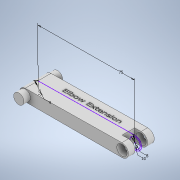
# Autodesk Inventor part: Elbow extension
Saved by Autodesk Inventor 2020 (Build 240168000, 168)
## iProperties
Created: 2020-12-23
Part Number: Elbow extension
Material: Generic
Document SubType Name: Modeling
Designer: frost
Density: 1 g/cm^3
Appearance: Default
Author: frost
Autodesk Inventor part; units mm, degrees
ref_plane "YZ Plane" through (0, 0, 0) normal (1, 0, 0) x (0, 1, 0)
ref_plane "XZ Plane" through (0, 0, 0) normal (0, 1, 0) x (-1, 0, 0)
ref_plane "XY Plane" through (0, 0, 0) normal (0, 0, 1) x (1, 0, 0)
sketch "Sketch1" plane through (0, 0, 0) normal (0, 0, 1) x (1, 0, 0)
  circle A0 centre (0, 0) radius 4
  circle A1 centre (74.9981, 0.5286) radius 4
  arc A2 (-0.0617, 4.4996) -> (0.0017, -4.5) centre (0, 0) ccw
  arc A3 (75, -4.4714) -> (74.9296, 5.5281) centre (74.9981, 0.5286) ccw
  line L0 (-0.0617, 4.4996) -> (74.9296, 5.5281)
  line L1 (0.0017, -4.5) -> (75, -4.4714)
  dimension "d0" = 8
  dimension "d1" = 8
  dimension "d2" = 75
  dimension "d3" = 9
  dimension "d4" = 10
  constraints: 4 centre point, 4 end point, 4 point on circle, 4 tangent, 3 coincident
  measures "d0" diameter of A0
  measures "d1" diameter of A1
  measures "d2" distance of A1.centre A0.centre
  measures "d3" diameter of A2
  measures "d4" diameter of A3
extrude "Extrusion1" add sketch "Sketch1" along normal mid plane 20 contours A0 | A1 | L0 A3 L1 A2
extrude "Extrusion2" add sketch "Sketch1" along normal mid plane 30 contours A0
extrude "Extrusion3" cut sketch "Sketch1" along normal mid plane 30 contours A1
sketch "Sketch2" plane through (-0.0617, 4.4996, 10) normal (-0.0137142, 0.999906, 0) x (0.999906, 0.0137142, 0)
  line L0 (15.9596, 15.3498) -> (61.2005, 15.3498) construction
  line L1 (61.2005, 15.3498) -> (61.2005, 12.0996) construction
  line L2 (61.2005, 12.0996) -> (15.9596, 12.0996) construction
  line L3 (15.9596, 12.0996) -> (15.9596, 15.3498) construction
  line L4 (16.4243, 12.1638) -> (16.4243, 15.2138)
  line L5 (16.4243, 15.2138) -> (19.2865, 15.2138)
  line L6 (19.2865, 15.2138) -> (19.2865, 14.853)
  line L7 (19.2865, 14.853) -> (17.0323, 14.853)
  line L8 (17.0323, 14.853) -> (17.0323, 14.0176)
  line L9 (17.0323, 14.0176) -> (19.1332, 14.0176)
  line L10 (19.1332, 14.0176) -> (19.1332, 13.6567)
  line L11 (19.1332, 13.6567) -> (17.0323, 13.6567)
  line L12 (17.0323, 13.6567) -> (17.0323, 12.5247)
  line L13 (17.0323, 12.5247) -> (19.2865, 12.5247)
  line L14 (19.2865, 12.5247) -> (19.2865, 12.1638)
  line L15 (19.2865, 12.1638) -> (16.4243, 12.1638)
  line L16 (20.4976, 12.1638) -> (19.9192, 12.1638)
  line L17 (19.9192, 12.1638) -> (19.9192, 15.3498)
  line L18 (19.9192, 15.3498) -> (20.4976, 15.3498)
  line L19 (20.4976, 15.3498) -> (20.4976, 12.1638)
  spline S0 degree 2 poles (24.2248, 13.3453) (24.2248, 12.7842) (23.4067, 12.0996) (22.7937, 12.0996) knots 0 0 0 1 2 2 2
  spline S1 degree 2 poles (22.7937, 12.0996) (22.5144, 12.0996) (22.1165, 12.191) (21.9237, 12.2701) knots 0 0 0 1 2 2 2
  line L20 (21.9237, 12.2701) -> (21.8866, 12.1638)
  line L21 (21.8866, 12.1638) -> (21.3453, 12.1638)
  line L22 (21.3453, 12.1638) -> (21.3453, 15.3498)
  line L23 (21.3453, 15.3498) -> (21.9237, 15.3498)
  line L24 (21.9237, 15.3498) -> (21.9237, 14.2128)
  spline S2 degree 2 poles (21.9237, 14.2128) (22.1412, 14.3438) (22.6528, 14.5168) (22.9741, 14.5168) knots 0 0 0 1 2 2 2
  spline S3 degree 2 poles (22.9741, 14.5168) (23.555, 14.5168) (24.2248, 13.8965) (24.2248, 13.3453) knots 0 0 0 1 2 2 2
  spline S4 degree 2 poles (23.6291, 13.3156) (23.6291, 13.7259) (23.2534, 14.151) (22.8382, 14.151) knots 0 0 0 1 2 2 2
  spline S5 degree 2 poles (22.8382, 14.151) (22.6034, 14.151) (22.1214, 14.0027) (21.9237, 13.889) knots 0 0 0 1 2 2 2
  line L25 (21.9237, 13.889) -> (21.9237, 12.5766)
  spline S6 degree 2 poles (21.9237, 12.5766) (22.1412, 12.5049) (22.4798, 12.4456) (22.6825, 12.4456) knots 0 0 0 1 2 2 2
  spline S7 degree 2 poles (22.6825, 12.4456) (23.1249, 12.4456) (23.6291, 12.8633) (23.6291, 13.3156) knots 0 0 0 1 2 2 2
  spline S8 degree 2 poles (27.6455, 13.3082) (27.6455, 12.7298) (26.8101, 12.0996) (26.1156, 12.0996) knots 0 0 0 1 2 2 2
  spline S9 degree 2 poles (26.1156, 12.0996) (25.4013, 12.0996) (24.5807, 12.7496) (24.5807, 13.3082) knots 0 0 0 1 2 2 2
  spline S10 degree 2 poles (24.5807, 13.3082) (24.5807, 13.8816) (25.426, 14.5168) (26.1156, 14.5168) knots 0 0 0 1 2 2 2
  spline S11 degree 2 poles (26.1156, 14.5168) (26.8101, 14.5168) (27.6455, 13.8841) (27.6455, 13.3082) knots 0 0 0 1 2 2 2
  spline S12 degree 2 poles (27.0499, 13.3082) (27.0499, 13.7531) (26.5654, 14.1856) (26.1156, 14.1856) knots 0 0 0 1 2 2 2
  spline S13 degree 2 poles (26.1156, 14.1856) (25.6658, 14.1856) (25.1764, 13.7531) (25.1764, 13.3082) knots 0 0 0 1 2 2 2
  spline S14 degree 2 poles (25.1764, 13.3082) (25.1764, 12.8757) (25.6658, 12.4308) (26.1156, 12.4308) knots 0 0 0 1 2 2 2
  spline S15 degree 2 poles (26.1156, 12.4308) (26.5605, 12.4308) (27.0499, 12.8683) (27.0499, 13.3082) knots 0 0 0 1 2 2 2
  line L26 (32.401, 14.4526) -> (31.531, 12.1638)
  line L27 (31.531, 12.1638) -> (30.9971, 12.1638)
  line L28 (30.9971, 12.1638) -> (30.1567, 13.9286)
  line L29 (30.1567, 13.9286) -> (29.3238, 12.1638)
  line L30 (29.3238, 12.1638) -> (28.7924, 12.1638)
  line L31 (28.7924, 12.1638) -> (27.9125, 14.4526)
  line L32 (27.9125, 14.4526) -> (28.5131, 14.4526)
  line L33 (28.5131, 14.4526) -> (29.1211, 12.6804)
  line L34 (29.1211, 12.6804) -> (29.9343, 14.4526)
  line L35 (29.9343, 14.4526) -> (30.4113, 14.4526)
  line L36 (30.4113, 14.4526) -> (31.2492, 12.6804)
  line L37 (31.2492, 12.6804) -> (31.8201, 14.4526)
  line L38 (31.8201, 14.4526) -> (32.401, 14.4526)
  line L39 (34.922, 12.1638) -> (34.922, 15.2138)
  line L40 (34.922, 15.2138) -> (37.7842, 15.2138)
  line L41 (37.7842, 15.2138) -> (37.7842, 14.853)
  line L42 (37.7842, 14.853) -> (35.5301, 14.853)
  line L43 (35.5301, 14.853) -> (35.5301, 14.0176)
  line L44 (35.5301, 14.0176) -> (37.631, 14.0176)
  line L45 (37.631, 14.0176) -> (37.631, 13.6567)
  line L46 (37.631, 13.6567) -> (35.5301, 13.6567)
  line L47 (35.5301, 13.6567) -> (35.5301, 12.5247)
  line L48 (35.5301, 12.5247) -> (37.7842, 12.5247)
  line L49 (37.7842, 12.5247) -> (37.7842, 12.1638)
  line L50 (37.7842, 12.1638) -> (34.922, 12.1638)
  line L51 (41.0739, 12.1638) -> (40.3646, 12.1638)
  line L52 (40.3646, 12.1638) -> (39.5292, 13.0264)
  line L53 (39.5292, 13.0264) -> (38.6715, 12.1638)
  line L54 (38.6715, 12.1638) -> (38.0165, 12.1638)
  line L55 (38.0165, 12.1638) -> (39.2079, 13.2983)
  line L56 (39.2079, 13.2983) -> (38.0289, 14.4526)
  line L57 (38.0289, 14.4526) -> (38.7383, 14.4526)
  line L58 (38.7383, 14.4526) -> (39.5662, 13.5949)
  line L59 (39.5662, 13.5949) -> (40.419, 14.4526)
  line L60 (40.419, 14.4526) -> (41.0739, 14.4526)
  line L61 (41.0739, 14.4526) -> (39.89, 13.3255)
  line L62 (39.89, 13.3255) -> (41.0739, 12.1638)
  spline S16 degree 2 poles (42.5569, 12.1194) (42.0848, 12.1194) (41.5559, 12.4777) (41.5559, 12.8658) knots 0 0 0 1 2 2 2
  line L63 (41.5559, 12.8658) -> (41.5559, 14.1337)
  line L64 (41.5559, 14.1337) -> (41.1654, 14.1337)
  line L65 (41.1654, 14.1337) -> (41.1654, 14.4526)
  line L66 (41.1654, 14.4526) -> (41.5559, 14.4526)
  line L67 (41.5559, 14.4526) -> (41.5559, 15.11)
  line L68 (41.5559, 15.11) -> (42.1343, 15.11)
  line L69 (42.1343, 15.11) -> (42.1343, 14.4526)
  line L70 (42.1343, 14.4526) -> (43.1971, 14.4526)
  line L71 (43.1971, 14.4526) -> (43.1971, 14.1337)
  line L72 (43.1971, 14.1337) -> (42.1343, 14.1337)
  line L73 (42.1343, 14.1337) -> (42.1343, 13.0437)
  spline S17 degree 2 poles (42.1343, 13.0437) (42.1343, 12.8707) (42.1516, 12.6804) (42.2134, 12.5988) knots 0 0 0 1 2 2 2
  spline S18 degree 2 poles (42.2134, 12.5988) (42.2653, 12.5272) (42.5001, 12.4555) (42.7003, 12.4555) knots 0 0 0 1 2 2 2
  spline S19 degree 2 poles (42.7003, 12.4555) (42.8412, 12.4555) (43.1056, 12.5123) (43.1625, 12.5296) knots 0 0 0 1 2 2 2
  line L74 (43.1625, 12.5296) -> (43.1971, 12.5296)
  line L75 (43.1971, 12.5296) -> (43.1971, 12.1836)
  spline S20 degree 2 poles (43.1971, 12.1836) (43.034, 12.154) (42.7003, 12.1194) (42.5569, 12.1194) knots 0 0 0 1 2 2 2
  spline S21 degree 2 poles (45.1151, 12.1119) (44.2945, 12.1119) (43.3874, 12.7274) (43.3874, 13.2958) knots 0 0 0 1 2 2 2
  spline S22 degree 2 poles (43.3874, 13.2958) (43.3874, 13.8544) (44.2673, 14.5168) (44.9767, 14.5168) knots 0 0 0 1 2 2 2
  spline S23 degree 2 poles (44.9767, 14.5168) (45.2955, 14.5168) (45.7874, 14.3933) (45.9727, 14.2623) knots 0 0 0 1 2 2 2
  spline S24 degree 2 poles (45.9727, 14.2623) (46.1556, 14.1313) (46.3534, 13.7531) (46.3534, 13.4788) knots 0 0 0 1 2 2 2
  line L76 (46.3534, 13.4788) -> (46.3534, 13.2687)
  line L77 (46.3534, 13.2687) -> (43.9732, 13.2687)
  spline S25 degree 2 poles (43.9732, 13.2687) (43.9732, 12.8707) (44.5763, 12.4481) (45.1077, 12.4481) knots 0 0 0 1 2 2 2
  spline S26 degree 2 poles (45.1077, 12.4481) (45.298, 12.4481) (45.6638, 12.5049) (45.8121, 12.5494) knots 0 0 0 1 2 2 2
  spline S27 degree 2 poles (45.8121, 12.5494) (45.9703, 12.5988) (46.1853, 12.6854) (46.2545, 12.7249) knots 0 0 0 1 2 2 2
  line L78 (46.2545, 12.7249) -> (46.2891, 12.7249)
  line L79 (46.2891, 12.7249) -> (46.2891, 12.3047)
  spline S28 degree 2 poles (46.2891, 12.3047) (46.1878, 12.2775) (45.8862, 12.1984) (45.7676, 12.1762) knots 0 0 0 1 2 2 2
  spline S29 degree 2 poles (45.7676, 12.1762) (45.597, 12.1441) (45.3252, 12.1119) (45.1151, 12.1119) knots 0 0 0 1 2 2 2
  spline S30 degree 2 poles (45.7898, 13.5628) (45.7849, 13.7185) (45.686, 13.9459) (45.5921, 14.0225) knots 0 0 0 1 2 2 2
  spline S31 degree 2 poles (45.5921, 14.0225) (45.4908, 14.109) (45.1744, 14.2005) (44.9421, 14.2005) knots 0 0 0 1 2 2 2
  spline S32 degree 2 poles (44.9421, 14.2005) (44.7097, 14.2005) (44.3884, 14.109) (44.2549, 14.02) knots 0 0 0 1 2 2 2
  spline S33 degree 2 poles (44.2549, 14.02) (44.1264, 13.9286) (43.9905, 13.7086) (43.9732, 13.5628) knots 0 0 0 1 2 2 2
  line L80 (43.9732, 13.5628) -> (45.7898, 13.5628)
  line L81 (49.6357, 12.1638) -> (49.0573, 12.1638)
  line L82 (49.0573, 12.1638) -> (49.0573, 13.4689)
  spline S34 degree 2 poles (49.0573, 13.4689) (49.0573, 13.627) (49.0104, 13.8989) (48.9461, 13.9805) knots 0 0 0 1 2 2 2
  spline S35 degree 2 poles (48.9461, 13.9805) (48.8769, 14.067) (48.6248, 14.151) (48.4048, 14.151) knots 0 0 0 1 2 2 2
  spline S36 degree 2 poles (48.4048, 14.151) (48.1898, 14.151) (47.7325, 13.9978) (47.515, 13.8742) knots 0 0 0 1 2 2 2
  line L83 (47.515, 13.8742) -> (47.515, 12.1638)
  line L84 (47.515, 12.1638) -> (46.9367, 12.1638)
  line L85 (46.9367, 12.1638) -> (46.9367, 14.4526)
  line L86 (46.9367, 14.4526) -> (47.515, 14.4526)
  line L87 (47.515, 14.4526) -> (47.515, 14.198)
  spline S37 degree 2 poles (47.515, 14.198) (47.7721, 14.3537) (48.2763, 14.5168) (48.5581, 14.5168) knots 0 0 0 1 2 2 2
  spline S38 degree 2 poles (48.5581, 14.5168) (49.0647, 14.5168) (49.6357, 14.0719) (49.6357, 13.6493) knots 0 0 0 1 2 2 2
  line L88 (49.6357, 13.6493) -> (49.6357, 12.1638)
  spline S39 degree 2 poles (51.3757, 12.1095) (51.0322, 12.1095) (50.434, 12.233) (50.2363, 12.3023) knots 0 0 0 1 2 2 2
  line L89 (50.2363, 12.3023) -> (50.2363, 12.7348)
  line L90 (50.2363, 12.7348) -> (50.266, 12.7348)
  spline S40 degree 2 poles (50.266, 12.7348) (50.3401, 12.6952) (50.5403, 12.6013) (50.7059, 12.5494) knots 0 0 0 1 2 2 2
  spline S41 degree 2 poles (50.7059, 12.5494) (50.8542, 12.5025) (51.2052, 12.4332) (51.3955, 12.4332) knots 0 0 0 1 2 2 2
  spline S42 degree 2 poles (51.3955, 12.4332) (51.5339, 12.4332) (51.8478, 12.4753) (51.9244, 12.5099) knots 0 0 0 1 2 2 2
  spline S43 degree 2 poles (51.9244, 12.5099) (52.0332, 12.5568) (52.1271, 12.6631) (52.1271, 12.7694) knots 0 0 0 1 2 2 2
  spline S44 degree 2 poles (52.1271, 12.7694) (52.1271, 12.9078) (51.9022, 13.0462) (51.618, 13.0932) knots 0 0 0 1 2 2 2
  spline S45 degree 2 poles (51.618, 13.0932) (51.5067, 13.1129) (51.1508, 13.1624) (51, 13.1896) knots 0 0 0 1 2 2 2
  spline S46 degree 2 poles (51, 13.1896) (50.6071, 13.2662) (50.2511, 13.5826) (50.2511, 13.8099) knots 0 0 0 1 2 2 2
  spline S47 degree 2 poles (50.2511, 13.8099) (50.2511, 14.1189) (50.9506, 14.507) (51.5314, 14.507) knots 0 0 0 1 2 2 2
  spline S48 degree 2 poles (51.5314, 14.507) (51.8182, 14.507) (52.394, 14.413) (52.5918, 14.3414) knots 0 0 0 1 2 2 2
  line L91 (52.5918, 14.3414) -> (52.5918, 13.9286)
  line L92 (52.5918, 13.9286) -> (52.5621, 13.9286)
  spline S49 degree 2 poles (52.5621, 13.9286) (52.3397, 14.0472) (51.7959, 14.1832) (51.5216, 14.1832) knots 0 0 0 1 2 2 2
  spline S50 degree 2 poles (51.5216, 14.1832) (51.2348, 14.1832) (50.8419, 14.0225) (50.8419, 13.8619) knots 0 0 0 1 2 2 2
  spline S51 degree 2 poles (50.8419, 13.8619) (50.8419, 13.716) (51.0742, 13.5751) (51.3312, 13.5307) knots 0 0 0 1 2 2 2
  spline S52 degree 2 poles (51.3312, 13.5307) (51.4622, 13.5084) (51.7786, 13.4639) (51.9541, 13.4367) knots 0 0 0 1 2 2 2
  spline S53 degree 2 poles (51.9541, 13.4367) (52.3347, 13.3725) (52.7178, 13.0783) (52.7178, 12.8238) knots 0 0 0 1 2 2 2
  spline S54 degree 2 poles (52.7178, 12.8238) (52.7178, 12.6755) (52.5423, 12.4135) (52.3743, 12.3171) knots 0 0 0 1 2 2 2
  spline S55 degree 2 poles (52.3743, 12.3171) (52.1889, 12.2157) (51.7267, 12.1095) (51.3757, 12.1095) knots 0 0 0 1 2 2 2
  line L93 (53.8449, 12.1638) -> (53.2665, 12.1638)
  line L94 (53.2665, 12.1638) -> (53.2665, 14.4526)
  line L95 (53.2665, 14.4526) -> (53.8449, 14.4526)
  line L96 (53.8449, 14.4526) -> (53.8449, 12.1638)
  line L97 (53.8869, 14.8332) -> (53.2295, 14.8332)
  line L98 (53.2295, 14.8332) -> (53.2295, 15.2336)
  line L99 (53.2295, 15.2336) -> (53.8869, 15.2336)
  line L100 (53.8869, 15.2336) -> (53.8869, 14.8332)
  spline S56 degree 2 poles (57.5153, 13.3082) (57.5153, 12.7298) (56.6799, 12.0996) (55.9853, 12.0996) knots 0 0 0 1 2 2 2
  spline S57 degree 2 poles (55.9853, 12.0996) (55.271, 12.0996) (54.4504, 12.7496) (54.4504, 13.3082) knots 0 0 0 1 2 2 2
  spline S58 degree 2 poles (54.4504, 13.3082) (54.4504, 13.8816) (55.2957, 14.5168) (55.9853, 14.5168) knots 0 0 0 1 2 2 2
  spline S59 degree 2 poles (55.9853, 14.5168) (56.6799, 14.5168) (57.5153, 13.8841) (57.5153, 13.3082) knots 0 0 0 1 2 2 2
  spline S60 degree 2 poles (56.9196, 13.3082) (56.9196, 13.7531) (56.4352, 14.1856) (55.9853, 14.1856) knots 0 0 0 1 2 2 2
  spline S61 degree 2 poles (55.9853, 14.1856) (55.5355, 14.1856) (55.0461, 13.7531) (55.0461, 13.3082) knots 0 0 0 1 2 2 2
  spline S62 degree 2 poles (55.0461, 13.3082) (55.0461, 12.8757) (55.5355, 12.4308) (55.9853, 12.4308) knots 0 0 0 1 2 2 2
  spline S63 degree 2 poles (55.9853, 12.4308) (56.4302, 12.4308) (56.9196, 12.8683) (56.9196, 13.3082) knots 0 0 0 1 2 2 2
  line L101 (60.8075, 12.1638) -> (60.2291, 12.1638)
  line L102 (60.2291, 12.1638) -> (60.2291, 13.4689)
  spline S64 degree 2 poles (60.2291, 13.4689) (60.2291, 13.627) (60.1822, 13.8989) (60.1179, 13.9805) knots 0 0 0 1 2 2 2
  spline S65 degree 2 poles (60.1179, 13.9805) (60.0487, 14.067) (59.7966, 14.151) (59.5766, 14.151) knots 0 0 0 1 2 2 2
  spline S66 degree 2 poles (59.5766, 14.151) (59.3616, 14.151) (58.9043, 13.9978) (58.6868, 13.8742) knots 0 0 0 1 2 2 2
  line L103 (58.6868, 13.8742) -> (58.6868, 12.1638)
  line L104 (58.6868, 12.1638) -> (58.1085, 12.1638)
  line L105 (58.1085, 12.1638) -> (58.1085, 14.4526)
  line L106 (58.1085, 14.4526) -> (58.6868, 14.4526)
  line L107 (58.6868, 14.4526) -> (58.6868, 14.198)
  spline S67 degree 2 poles (58.6868, 14.198) (58.9439, 14.3537) (59.4481, 14.5168) (59.7299, 14.5168) knots 0 0 0 1 2 2 2
  spline S68 degree 2 poles (59.7299, 14.5168) (60.2365, 14.5168) (60.8075, 14.0719) (60.8075, 13.6493) knots 0 0 0 1 2 2 2
  line L108 (60.8075, 13.6493) -> (60.8075, 12.1638)
  point P0 (0, 10)
  constraints: 2 other
extrude "Extrusion4" cut sketch "Sketch2" against normal blind 5
sketch "Sketch3" plane through (-0.0617, 4.4996, 10) normal (-0.0137142, 0.999906, 0) x (0.999906, 0.0137142, 0)
  line L0 (73.82, 0.1058) -> (73.82, 5.1058)
  line L1 (79.9983, 20) -> (79.9983, 0) projected
  line L2 (79.9983, 5.1058) -> (69.9983, 5.1058)
  line L3 (79.9983, 5.1058) -> (89.9983, 5.1058) construction
  line L4 (74.9317, 20) -> (74.9317, 0) projected
  line L5 (74.9317, 10) -> (69.1306, 10)
  line L6 (79.9983, 14.8942) -> (69.9983, 14.8942)
  line L7 (69.9983, 5.1058) -> (69.9983, 14.8942)
  line L8 (79.9983, 5.1058) -> (79.9983, 14.8942)
  point P0 (0, 10)
  dimension "d13" = 5
  dimension "d14" = 10
  dimension "d15" = 180
  constraints: 14 end point, 3 vertical, 2 horizontal, 2 symmetric about line, 1 collinear, 1 midpoint, 1 perpendicular, 1 point on line
  measures "d13" distance of L0.start L0.end
  measures "d14" distance of L2.start L2.end
  measures "d15" angle of L2 L3
extrude "Extrusion5" cut sketch "Sketch3" against normal blind 10
body "Solid1"
